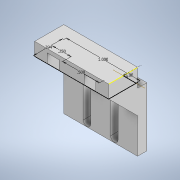
# Autodesk Inventor part: door limit switch holder
Saved by Autodesk Inventor 2020 (Build 240168000, 168)
## iProperties
Created: 2022-02-13
Part Number: door limit switch holder
Material: Generic
Document SubType Name: Modeling
Designer: Beaucage
Density: 1 g/cm^3
Appearance: Default
Author: Beaucage
Autodesk Inventor part; units mm, degrees
ref_plane "YZ Plane" through (0, 0, 0) normal (1, 0, 0) x (0, 1, 0)
ref_plane "XZ Plane" through (0, 0, 0) normal (0, 1, 0) x (-1, 0, 0)
ref_plane "XY Plane" through (0, 0, 0) normal (0, 0, 1) x (1, 0, 0)
sketch "Sketch1" plane through (0, 0, 0) normal (0, 1, 0) x (-1, 0, 0)
  line L0 (0, 0) -> (25.4, 0)
  line L1 (25.4, 0) -> (25.4, -10)
  line L2 (25.4, -10) -> (0, -10)
  line L3 (0, -10) -> (0, 0)
  line L4 (25.4, -5) -> (19.05, -5)
  line L5 (19.05, -5) -> (6.35, -5)
  dimension "d0" = 25.4
  dimension "d1" = 10
  dimension "d4" = 6.35
  dimension "d5" = 12.7
  constraints: 12 end point, 2 horizontal, 2 parallel, 1 midpoint, 1 perpendicular, 1 point on line
  measures "d0" distance of L1.end L2.end
  measures "d1" distance of L0.end L1.end
  measures "d4" distance of L4.start L4.end
  measures "d5" distance of L4.end L5.end
extrude "Extrusion1" add sketch "Sketch1" along normal blind 4.445
hole "Hole1" at (-6.35, 0, -5) at (-19.05, 0, -5) direction (0, 1, 0) diameter 10.795 depth 3.175
sketch "Sketch2" plane through (0, 0, 0) normal (0, -1, 0) x (1, 0, 0)
  line L0 (-25.4, 0) -> (0, 0) projected
  line L1 (0, -10) -> (-25.4, -10) projected
  line L2 (0, 0) -> (-0.635, 0)
  line L3 (-0.635, 0) -> (-0.635, -10)
  line L4 (-0.635, -10) -> (0, -10)
  line L5 (0, -10) -> (0, 0)
  line L6 (-17.017, 0) -> (-8.383, 0) projected
  line L7 (-12.7, 0) -> (-12.0585, 0)
  line L8 (-12.0585, 0) -> (-12.0585, -10)
  line L9 (-12.0585, -10) -> (-12.7, -10)
  line L10 (-12.7, -10) -> (-12.7, 0)
  line L11 (-12.7, -10) -> (-13.3295, -10)
  line L12 (-13.3295, -10) -> (-13.3295, 0)
  line L13 (-13.3295, 0) -> (-12.7, 0)
  line L14 (-12.7, 0) -> (-12.7, -10)
  line L15 (-25.4, -10) -> (-25.4, 0) projected
  line L16 (-25.4, 0) -> (-21.083, 0) projected
  line L17 (-25.4, -10) -> (-24.765, -10)
  line L18 (-24.765, -10) -> (-24.765, 0)
  line L19 (-24.765, 0) -> (-25.4, 0)
  line L20 (-25.4, 0) -> (-25.4, -10)
  point P0 (-24.765, 0)
  dimension "d13" = 0.635
  dimension "d14" = 0.635
  constraints: 32 end point, 8 parallel, 4 horizontal, 4 perpendicular, 4 point on line, 1 midpoint
  measures "d13" distance of L4.end L3.end
  measures "d14" distance of L19.end L18.end
sketch "Sketch3" plane through (0, 0, 0) normal (1, 0, 0) x (0, 0, -1)
  line L0 (0, 4.445) -> (10, 4.445) projected
  line L1 (5, 4.445) -> (9.445, 0)
  line L2 (10, 0) -> (0, 0) projected
  line L3 (5, 4.445) -> (11.2862, 4.445) construction
  dimension "d15" = 45
  constraints: 4 end point, 1 equal length, 1 horizontal, 1 midpoint, 1 point on line
  measures "d15" angle of L1 L3
extrude "Extrusion2" add sketch "Sketch2" along normal blind 25.4 contours L0 L18 L1 L15 | L12 L0 L10 L1 | L10 L0 L8 L1 | L3 L0 L5 L1
sketch "Sketch4" plane through (0, 4.445, 0) normal (1, 0, 0) x (0, 0, -1)
  line L0 (0, -4.445) -> (10, -14.445)
  line L1 (10, -29.845) -> (10, 0) projected
  line L2 (0, -4.445) -> (14.1421, -4.445) construction
  line L3 (0, -4.445) -> (0, -29.845) projected
  line L4 (0, -4.445) -> (0, -29.845)
  line L5 (0, -29.845) -> (10, -29.845) projected
  line L6 (0, -29.845) -> (10, -29.845)
  line L7 (10, -29.845) -> (10, -14.445)
  dimension "d18" = 45
  constraints: 10 end point, 2 perpendicular, 1 equal length, 1 horizontal, 1 point on line, 1 vertical
  measures "d18" angle of L0 L2
extrude "Extrusion3" cut sketch "Sketch4" against normal blind 25.4
sketch "Sketch5" plane through (0, 4.445, -10) normal (0, 0, -1) x (-1, 0, 0)
  line L0 (25.4, -14.445) -> (25.4, -4.445) projected
  line L1 (-13.6769, -18.89) -> (25.4, -18.89)
  line L2 (25.4, -18.89) -> (25.4, -6.19)
  line L3 (25.4, -6.19) -> (-13.6769, -6.19)
  line L4 (-13.6769, -6.19) -> (-13.6769, -18.89)
  line L5 (0, -14.445) -> (0, 0) projected
  line L6 (0, -6.19) -> (25.4, -6.19)
  line L7 (25.4, -6.19) -> (25.4, -26.51)
  line L8 (25.4, -26.51) -> (0, -26.51)
  line L9 (0, -26.51) -> (0, -6.19)
  point P0 (0, -4.445)
  point P1 (25.4, -18.89)
  dimension "d21" = 12.7
  dimension "d28" = 20.32
  constraints: 16 end point, 4 parallel, 3 point on line, 2 horizontal, 2 perpendicular
  measures "d21" distance of L2.end L1.end
  measures "d28" distance of L6.end L7.end
extrude "Extrusion4" add sketch "Sketch5" along normal blind 3.175 contours L2 L1 L9 L5 L3 L0 | L7 L8 L9 L1
sketch "Sketch6" plane through (0, 4.445, -13.175) normal (0, 0, -1) x (-1, 0, 0)
  line L0 (12.0585, -6.19) -> (13.3295, -6.19) projected
  line L1 (12.694, -6.19) -> (12.694, -11.3085)
  line L2 (12.694, -11.3085) -> (12.694, -19.0349)
  line L3 (12.694, -16.1482) -> (7.995, -16.1482)
  line L4 (7.995, -16.1482) -> (17.393, -16.1482)
  line L5 (7.995, -21.2233) -> (7.995, -11.0732) construction
  line L6 (9.265, -21.2233) -> (9.265, -11.0732)
  line L7 (6.725, -11.0732) -> (6.725, -21.2233)
  arc A0 (6.725, -21.2233) -> (9.265, -21.2233) centre (7.995, -21.2233) ccw
  arc A1 (9.265, -11.0732) -> (6.725, -11.0732) centre (7.995, -11.0732) ccw
  line L8 (17.393, -21.2233) -> (17.393, -11.0732) construction
  line L9 (18.663, -21.2233) -> (18.663, -11.0732)
  line L10 (16.123, -11.0732) -> (16.123, -21.2233)
  arc A2 (16.123, -21.2233) -> (18.663, -21.2233) centre (17.393, -21.2233) ccw
  arc A3 (18.663, -11.0732) -> (16.123, -11.0732) centre (17.393, -11.0732) ccw
  line L11 (7.995, -25.0382) -> (7.995, -7.2582) construction
  line L12 (9.265, -25.0382) -> (9.265, -7.2582)
  line L13 (6.725, -7.2582) -> (6.725, -25.0382)
  arc A4 (6.725, -25.0382) -> (9.265, -25.0382) centre (7.995, -25.0382) ccw
  arc A5 (9.265, -7.2582) -> (6.725, -7.2582) centre (7.995, -7.2582) ccw
  line L14 (17.393, -25.0382) -> (17.393, -7.2582) construction
  line L15 (18.663, -25.0382) -> (18.663, -7.2582)
  line L16 (16.123, -7.2582) -> (16.123, -25.0382)
  arc A6 (16.123, -25.0382) -> (18.663, -25.0382) centre (17.393, -25.0382) ccw
  arc A7 (18.663, -7.2582) -> (16.123, -7.2582) centre (17.393, -7.2582) ccw
  point P0 (0, -4.445)
  point P1 (18.663, -11.0732)
  dimension "d24" = 4.699
  dimension "d25" = 9.398
  dimension "d26" = 2.54
  dimension "d27" = 2.54
  dimension "d29" = 8.89
  dimension "d30" = 2.54
  dimension "d31" = 8.89
  dimension "d32" = 2.54
  constraints: 40 end point, 16 point on circle, 16 tangent, 8 centre point, 5 midpoint, 5 point on line, 4 parallel, 2 vertical, 1 perpendicular
  measures "d24" distance of L3.start L3.end
  measures "d25" distance of L3.end L4.end
  measures "d26" diameter of A1
  measures "d27" diameter of A3
  measures "d29" distance of L3.end L11.end
  measures "d30" diameter of A5
  measures "d31" distance of L4.end L14.end
  measures "d32" diameter of A7
extrude "Extrusion5" cut sketch "Sketch6" against normal blind 3.175
body "Solid1"
